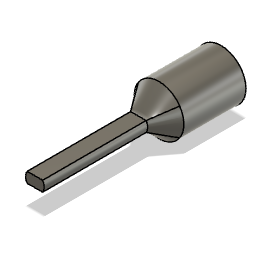
Coupleur (ancien moteur) (Autodesk Fusion 360 design; units mm, degrees)
Autodesk Fusion 360 part; units mm, degrees
note: some values were not read from the file. Set by a fixed rule: which sketch regions a step uses.
sketch "Esquisse1" plane through (0, 0, 0) normal (0, 0, 1) x (1, 0, 0)
  circle A0 centre (0, 0) radius 3.5
  circle A1 centre (0, 0) radius 6
  line L0 (1.8028, -3) -> (-1.8028, -3)
  line L1 (-1.8028, -3) -> (-1.8028, -3.5)
  line L2 (-1.8028, -3.5) -> (1.8028, -3.5)
  line L3 (1.8028, -3.5) -> (1.8028, -3)
  dimension "d1" = 7
  dimension "d2" = 12
  dimension "d17" = 0.5
  constraint coincident A0.centre A1.centre
  constraint concentric A0 A1
  constraint horizontal L0
  constraint vertical L1
  constraint horizontal L2
  constraint vertical L3
  constraint coincident A0 L0.start
  constraint coincident A0 L0.end
  constraint tangent A0 L2
  measures "d1" diameter of A0
  measures "d2" diameter of A1
  measures "d17" distance of L0.start L2.end
extrude "Extrusion1" add sketch "Esquisse1" along normal blind 15 contours A0 L0 | A0 L1 L2 | A0 L2 L3 | A1 picked at (0.4606, -3.0719)
ref_plane "Plan de construction1" through (0, 0, 20) normal (0, 0, 1) x (1, 0, 0)
sketch "Esquisse2" plane through (0, 0, 20) normal (0, 0, 1) x (1, 0, 0)
  line L0 (-1.8708, 1.25) -> (1.8708, 1.25)
  line L1 (1.8708, -1.25) -> (-1.8708, -1.25)
  arc A0 (-1.8708, 1.25) -> (-1.8708, -1.25) centre (0, 0) ccw
  arc A1 (1.8708, -1.25) -> (1.8708, 1.25) centre (0, 0) ccw
  dimension "d6" = 4.5
  dimension "d16" = 2.5
  constraint coincident A0.centre A1.centre
  constraint parallel L0 L1
  constraint coincident L1.start A0
  constraint concentric A0 A1
  constraint horizontal L0
  constraint equal L0 L1
  measures "d6" diameter of A0
  measures "d16" distance of L0 L1
sketch "Esquisse3" plane through (0, 0, 15) normal (0, 0, 1) x (1, 0, 0)
  circle A0 centre (0, 0) radius 6
  circle A1 centre (0, 0) radius 6
  arc A2 (1.8028, -3) -> (-1.8028, -3) centre (0, 0) ccw
  line L0 (1.8028, -3) -> (-1.8028, -3)
  dimension "d13" = 12
  constraint concentric A1 A2
  measures "d13" diameter of A1
loft "Lissage1" add profiles "Esquisse3", "Esquisse2" section 1 contours A0 A1 | A2 L0 section 2
extrude "Extrusion2" add 1 faces at (0.6236, -0.4167, 20) along direction (0, 0, 1) blind 25
sketch "Esquisse4" plane through (0, 0, 0) normal (0, 1, 0) x (1, 0, 0)
  circle A0 centre (0, -5) radius 1.5
  line L0 (0, 0) -> (0, -15) construction
  line L1 (-4.9889, -15) -> (4.9889, -15)
  dimension "d11" = 3
  dimension "d12" = 5
  constraint coincident L0.start origin
  constraint vertical L0
  constraint coincident A0.centre L0
  constraint coincident L0.end L1
  measures "d11" diameter of A0
  measures "d12" vertical distance of L0.start A0.centre
extrude "Extrusion3" cut sketch "Esquisse4" against normal blind 10
equation "d9 = 5 mm + 3 mm + 5 mm + 5 mm + 7 mm"
